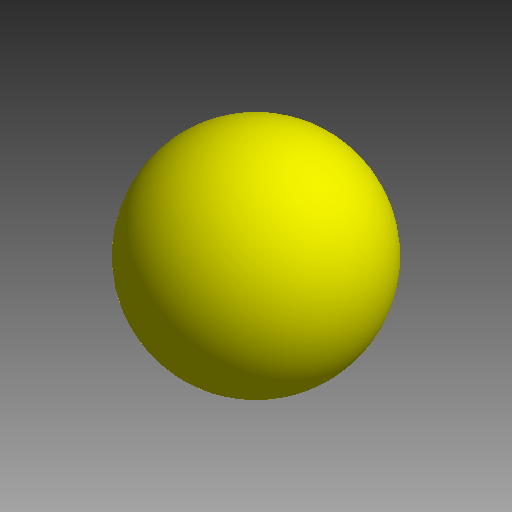
# Autodesk Inventor part: W 638/3-2Z_PART3
Saved by Autodesk Inventor 2018 (Build 220112000, 112)
## iProperties
Category: PARTsolutions
Company: SKF
Part Number: W 638/3-2Z_PART3
Material: Generic
Catalog Web Link: www.cadenas.de
Description: -Deep groove ball bearings
Vendor: SKF
Document SubType Name: Modeling
Designer: partserver
Manufacturer: SKF
Mass: 0.000523599 g
Surface Area: 0.0314159 cm^2
Volume: 0.000523599 cm^3
Density: 1 g/cm^3
Appearance: PSOLRGB-192-192-192
PSOL_IDENT_0: {$CADENAS_DATA\23d-libs\skf_r32\bearings_units_and_housings\ball_bearings\deep_groove_ball_bearings\
PSOL_IDENT_1: bb1_001_101.prj},199 {VTYP=3D},{NB=W 638/3-2Z_PART3},{LINA=W 638/3-2Z_PART3},{NN=BB1_001_101_PART3},
PSOL_IDENT_2: {NOPRJ=TRUE},{DATE=03.04.2020 14:22:31},{GEOMDATE=30.03.2020 16:10:03},{VERSION=},{LINEID=19220},{WB
PSOL_IDENT_3: VAR=},{WBNUMERIC=}  {NB=W 638/3-2Z_PART3},{LINA=W 638/3-2Z_PART3},{KT=DUMMY},{DESIGNATION=W 638/3-2Z
PSOL_IDENT_4: },{DD=3.000},{D=7.000},{B=3.000},{C=0.000},{DD1=0.00},{DD2=3.90},{D1=0.00},{D2=6.35},{D3=0.000},{D4=
PSOL_IDENT_5: 0.000},{HH=MIN},{BB=0.000},{FF=0.00},{R0MAX=MIN},{R0=MIN},{R12=0.10},{PITCH=5.00},{DW=1.000},{DDAMIN=
PSOL_IDENT_6: 3.700},{DDAMAX=3.800},{DDBMIN=MIN},{DDBMAX=MIN},{DBMIN=MIN},{DAMAX=6.500},{BBAMIN=MIN},{CAMAX=MIN},{
PSOL_IDENT_7: RAMAX=0.100},{LOAD1=0.178},{LOAD2=0.057},{LOAD3=0.002},{SPEED1=160000},{SPEED2=80000},{KR=0.020},{F0=
PSOL_IDENT_8: 7.100},{Z=8},{II=1},{MASS=0.000},{BEARING=W 638/3-2Z},{RING=},{HELP=0.665},{HELP2=0.325},{DD1ALG=2.0
PSOL_IDENT_9: 00},{YALG=2.175},{PITCH1=5.000},{DW1=1.000},{YALG1=2.835},{HALG1=0.665},{SH=1.950},{CU=0.400},{DESIG
PSOL_IDENT_10: N=dgbbw2z},{HALG=0.675},{B1=0},{SHIELDHELP=2}
NB: W 638/3-2Z_PART3
NT: Deep groove ball bearings
NBSYN: $DESIGNATION._PART3
LINA: W 638/3-2Z_PART3
CATALOG: SKF
SUPPLIER: SKF
ARTICLENO: W 638/3-2Z_PART3
BOMINFO: W 638/3-2Z_PART3
CREATOR: CADENAS GmbH
Title: W 638/3-2Z_PART3
Author: Cadenas PARTsolutions
Comments: Deep groove ball bearings
Autodesk Inventor part; units mm, degrees
ref_plane "YZ Plane" through (0, 0, 0) normal (1, 0, 0) x (0, 1, 0)
ref_plane "XZ Plane" through (0, 0, 0) normal (0, 1, 0) x (-1, 0, 0)
ref_plane "XY Plane" through (0, 0, 0) normal (0, 0, 1) x (1, 0, 0)
sketch "Sketch_6" plane through (0, 0, 0) normal (0, 0, 1) x (1, 0, 0)
  line L0 (2, 2.5) -> (1, 2.5)
  arc A0 (2, 2.5) -> (1, 2.5) centre (1.5, 2.5) ccw
  line L1 (2, 2.5) -> (1, 2.5)
  dimension "d0" = 360
  constraints: 4 end point, 2 point on circle, 1 centre point
revolve "Revolution1" add sketch "Sketch_6" angle 360 about axis through (2, 2.5, 0) along (1, 0, 0)
body "Solid1"
